# Autodesk Inventor part: JUMPER-PAD-2-NOYES_SILK
Saved by Autodesk Inventor 2016 SP1 (Build 200210100, 210)
## iProperties
Created: 2015-11-19
Part Number: JUMPER-PAD-2-NOYES_SILK
Material: Generic
Document SubType Name: Modeling
Designer: PhillipD
Density: 1 g/cm^3
Appearance: PAD-JUMPER-2-NO_YES_SILK, JUMPER-PAD-2-NOYES_SILK
Author: PhillipD
Autodesk Inventor part; units mm, degrees
ref_plane "YZ Plane" through (0, 0, 0) normal (1, 0, 0) x (0, 1, 0)
ref_plane "XZ Plane" through (0, 0, 0) normal (0, 1, 0) x (-1, 0, 0)
ref_plane "XY Plane" through (0, 0, 0) normal (0, 0, 1) x (1, 0, 0)
sketch "PAD-JUMPER-2-NO_YES_SILK, JUMPER-PAD-2-NOYES_SILK_54" plane through (0, 0, 0) normal (0, 0, 1) x (1, 0, 0)
  line L0 (-1.1065, 1) -> (1.005, 1)
  line L1 (1.005, 1) -> (1.005, -1.1016)
  line L2 (1.005, -1.1016) -> (-1.1065, -1.1016)
  line L3 (-1.1065, -1.1016) -> (-1.1065, 1)
  constraints: 8 end point
extrude "Extrusion1" add sketch "PAD-JUMPER-2-NO_YES_SILK, JUMPER-PAD-2-NOYES_SILK_54" along normal blind 1
body "Solid1"
